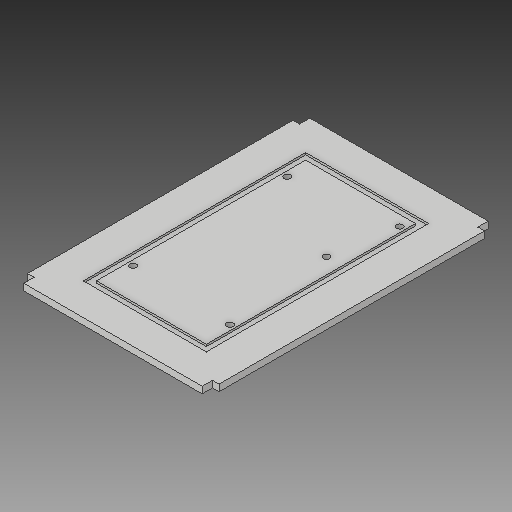
# Autodesk Inventor part: Cuerpo - Base Arduino
Saved by Autodesk Inventor 2019 (Build 230136000, 136)
## iProperties
Created: 2020-03-13
Part Number: Cuerpo - Base Arduino
Material: Generic
Document SubType Name: Modeling
Designer: Sanoli
Density: 1 g/cm^3
Appearance: Default
Author: Sanoli
Autodesk Inventor part; units mm, degrees
ref_plane "YZ Plane" through (0, 0, 0) normal (1, 0, 0) x (0, 1, 0)
ref_plane "XZ Plane" through (0, 0, 0) normal (0, 1, 0) x (-1, 0, 0)
ref_plane "XY Plane" through (0, 0, 0) normal (0, 0, 1) x (1, 0, 0)
sketch "Sketch1" plane through (0, 0, 0) normal (0, 1, 0) x (-1, 0, 0)
  line L0 (0, 0) -> (93.0623, 0)
  line L1 (93.0623, 0) -> (93.0623, -128.95)
  line L2 (93.0623, -128.95) -> (0, -128.95)
  line L3 (0, -128.95) -> (0, 0)
  dimension "d0" = 93.0623
  dimension "d1" = 128.95
  constraints: 8 end point, 2 parallel, 1 horizontal, 1 perpendicular
  measures "d0" distance of L1.end L2.end
  measures "d1" distance of L0.end L1.end
extrude "Extrusion1" add sketch "Sketch1" along normal blind 3.2
sketch "Sketch2" plane through (0, 3.2, 0) normal (0, 1, 0) x (1, 0, 0)
  line L0 (-73.2061, 115.27) -> (-19.8561, 115.27)
  line L1 (-19.8561, 115.27) -> (-19.8561, 13.68)
  line L2 (-19.8561, 13.68) -> (-73.2061, 13.68)
  line L3 (-73.2061, 13.68) -> (-73.2061, 115.27)
  circle A0 centre (-70.6561, 28.92) radius 1.5875
  circle A1 centre (-22.3961, 27.65) radius 1.5875
  circle A2 centre (-22.3961, 110.2) radius 1.5875
  circle A3 centre (-70.6561, 103.85) radius 1.5875
  circle A4 centre (-27.4761, 79.72) radius 1.5875
  line L4 (-93.0623, 0) -> (0, 0) projected
  line L5 (-93.0623, 128.95) -> (-93.0623, 0) projected
  line L6 (0, 128.95) -> (-93.0623, 128.95) projected
  line L7 (-76.4061, 118.47) -> (-16.6561, 118.47)
  line L8 (-16.6561, 118.47) -> (-16.6561, 10.48)
  line L9 (-16.6561, 10.48) -> (-76.4061, 10.48)
  line L10 (-76.4061, 10.48) -> (-76.4061, 118.47)
  dimension "d4" = 101.59
  dimension "d5" = 53.35
  dimension "d6" = 15.24
  dimension "d7" = 3.175
  dimension "d8" = 50.8
  dimension "d9" = 13.97
  dimension "d10" = 2.54
  dimension "d11" = 90.17
  dimension "d12" = 96.52
  dimension "d13" = 50.8
  dimension "d14" = 2.54
  dimension "d15" = 66.04
  dimension "d16" = 7.62
  dimension "d20" = 93.0623
  dimension "d21" = 19.8561
  dimension "d22" = 128.95
  dimension "d23" = 13.68
  dimension "d26" = 3.2
  dimension "d27" = 3.2
  dimension "d28" = 3.2
  dimension "d29" = 3.2
  constraints: 16 end point, 5 centre point, 4 equal radius, 4 parallel, 2 horizontal, 2 perpendicular
  measures "d4" distance of L0.end L1.end
  measures "d5" distance of L1.end L2.end
  measures "d6" distance from line of L2 A0.centre
  measures "d7" diameter of A0
  measures "d8" distance from line of A0.centre L1
  measures "d9" distance from line of L2 A1.centre
  measures "d10" distance from line of A1.centre L1
  measures "d11" distance from line of A3.centre L2
  measures "d12" distance from line of A2.centre L2
  measures "d13" distance from line of A3.centre L1
  measures "d14" distance from line of A2.centre L1
  measures "d15" distance from line of A4.centre L2
  measures "d16" distance from line of A4.centre L1
  measures "d20" distance of L6.start L5.start
  measures "d21" distance between parallel lines of L5 L3
  measures "d22" distance of L5.start L4.start
  measures "d23" distance between parallel lines of L4 L2
  measures "d26" distance between parallel lines of L0 L7
  measures "d27" distance between parallel lines of L10 L3
  measures "d28" distance between parallel lines of L8 L1
  measures "d29" distance between parallel lines of L2 L9
extrude "Extrusion2" cut sketch "Sketch2" against normal up to surface (3.2 mm away) contours A0 | A1 | A2 | A3 | A4
sketch "Sketch3" plane through (0, 3.2, 0) normal (0, 1, 0) x (1, 0, 0)
  line L0 (-76.4061, 10.48) -> (-76.4061, 118.47) projected
  line L1 (-73.2061, 13.68) -> (-73.2061, 115.27) projected
  line L2 (-19.8561, 13.68) -> (-73.2061, 13.68) projected
  line L3 (-16.6561, 10.48) -> (-76.4061, 10.48) projected
  line L4 (-16.6561, 118.47) -> (-16.6561, 10.48) projected
  line L5 (-73.2061, 115.27) -> (-19.8561, 115.27) projected
  line L6 (-76.4061, 118.47) -> (-16.6561, 118.47) projected
  line L7 (-19.8561, 115.27) -> (-19.8561, 13.68) projected
  point P0 (0, 0)
extrude "Extrusion3" cut sketch "Sketch3" against normal blind 1
sketch "Sketch4" plane through (0, 3.2, 0) normal (0, 1, 0) x (1, 0, 0)
  line L0 (-93.0623, 0) -> (0, 0) projected
  line L1 (-89.8623, 0) -> (-3.2, 0)
  line L2 (-3.2, 0) -> (-3.2, -5)
  line L3 (-3.2, -5) -> (-89.8623, -5)
  line L4 (-89.8623, -5) -> (-89.8623, 0)
  line L5 (0, 128.95) -> (-93.0623, 128.95) projected
  line L6 (-89.8623, 128.95) -> (-3.2, 128.95)
  line L7 (-3.2, 128.95) -> (-3.2, 133.95)
  line L8 (-3.2, 133.95) -> (-89.8623, 133.95)
  line L9 (-89.8623, 133.95) -> (-89.8623, 128.95)
  line L10 (-93.0623, 128.95) -> (-93.0623, 0) projected
  line L11 (0, 0) -> (0, 128.95) projected
  dimension "d32" = 3.2
  dimension "d33" = 3.2
  dimension "d34" = 5
  dimension "d35" = 5
  constraints: 16 end point, 4 parallel, 4 point on line, 2 horizontal, 2 perpendicular
  measures "d32" distance between parallel lines of L10 L4
  measures "d33" distance between parallel lines of L11 L2
  measures "d34" distance between parallel lines of L0 L3
  measures "d35" distance between parallel lines of L5 L8
extrude "Extrusion4" add sketch "Sketch4" against normal up to surface (3.2 mm away) contours L0 L2 L3 L4 | L9 L8 L7 L5
equation "\"d1\" = largo_abdomen_robot - acople_hombro_grosor_trasero"
equation "\"d13\" = d8"
equation "\"d14\" = d10"
equation "\"d21\" = -0.5 * d5 + 0.5 * d20"
equation "\"d23\" = -0.5 * d4 + 0.5 * d22"
equation "\"d27\" = d26"
equation "\"d28\" = d26"
equation "\"d29\" = d28"
equation "\"d33\" = d32"
equation "\"d35\" = d34"
equation "\"largo_abdomen_robot\" = 146.95"
equation "\"acople_hombro_grosor_trasero\" = 18"
body "Solid1"
